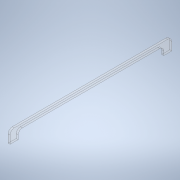
# Autodesk Inventor part: IndexRailM
Saved by Autodesk Inventor 2022 (Build 260153000, 153)
## iProperties
Created: 2022-01-13
Part Number: IndexRailM
Material: Polycarbonate, Clear
Document SubType Name: Modeling
Designer: tagaz
Density: 1.2 g/cm^3
Appearance: Polycarbonate - Clear
Author: tagaz
Autodesk Inventor part; units mm, degrees
ref_plane "YZ Plane" through (0, 0, 0) normal (1, 0, 0) x (0, 1, 0)
ref_plane "XZ Plane" through (0, 0, 0) normal (0, 1, 0) x (-1, 0, 0)
ref_plane "XY Plane" through (0, 0, 0) normal (0, 0, 1) x (1, 0, 0)
sketch "Sketch1" plane through (0, 0, 0) normal (1, 0, 0) x (0, 1, 0)
  line L0 (0, 0) -> (12.7, 0)
  line L1 (38.1, 0) -> (38.1, 12.7)
  line L2 (25.4, 25.4) -> (0, 25.4)
  line L3 (0, 25.4) -> (0, 0)
  line L4 (25.4, -12.7) -> (25.4, -444.5)
  line L5 (38.1, -469.9) -> (38.1, 12.7)
  line L6 (25.4, -482.6) -> (0, -482.6)
  line L7 (0, -482.6) -> (0, -457.2)
  line L8 (0, -457.2) -> (12.7, -457.2)
  line L9 (38.1, -457.2) -> (38.1, -469.9)
  arc A0 (38.1, 12.7) -> (25.4, 25.4) centre (25.4, 12.7) ccw
  arc A1 (25.4, -12.7) -> (12.7, 0) centre (12.7, -12.7) ccw
  arc A2 (12.7, -457.2) -> (25.4, -444.5) centre (12.7, -444.5) ccw
  arc A3 (25.4, -482.6) -> (38.1, -469.9) centre (25.4, -469.9) ccw
  dimension "d4" = 38.1
  dimension "d5" = 25.4
  dimension "d6" = 12.7
  dimension "d7" = 12.7
  dimension "d8" = 12.7
  dimension "d9" = 508
  dimension "d10" = 25.4
  dimension "d11" = 38.1
  dimension "d12" = 38.1
  constraints: 20 end point, 8 point on circle, 8 tangent, 5 parallel, 4 centre point, 2 equal radius, 2 horizontal, 2 perpendicular
  measures "d4" distance of L7.end L9.start
  measures "d5" distance of L6.end L7.end
  measures "d6" radius of A0
  measures "d7" radius of A1
  measures "d8" distance between parallel lines of L4 L5
  measures "d9" distance between parallel lines of L2 L6
  measures "d10" distance between parallel lines of L0 L2
  measures "d11" distance between parallel lines of L5 L3
  measures "d12" distance between parallel lines of L9 L7
extrude "Extrusion1" add sketch "Sketch1" along normal blind 6.35
body "Solid1"
